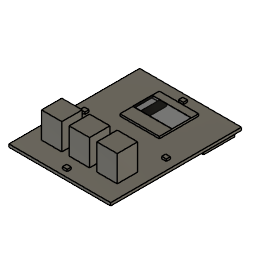
Telemetry Assembly (Autodesk Fusion 360 archive; units mm, degrees)
design "Telemetry PCB"
part number: 2026-03-18-11-21-59-184
Autodesk Fusion 360 part; units mm, degrees
sketch "Sketch1" plane through (0, 0, 0) normal (0, 0, 1) x (1, 0, 0)
  line L0 (-55, 55) -> (15, 55)
  line L1 (15, 55) -> (15, -35)
  line L2 (15, -35) -> (-55, -35)
  line L3 (-55, -35) -> (-55, 55)
  dimension "d1" = 70
  dimension "d2" = 90
  constraint horizontal L0
  constraint vertical L1
  constraint horizontal L2
  constraint vertical L3
  measures "d1" distance of L0.start L0.end
  measures "d2" distance of L0.start L2.end
extrude "Extrude1" add sketch "Sketch1" along normal blind 2 makes body 1
sketch "Display" plane through (0, 0, 2) normal (0, 0, 1) x (-1, 0, 0)
  line L0 (55, 35) -> (-15, 35)
  line L1 (-15, 35) -> (-15, -55)
  line L2 (-15, -55) -> (55, -55)
  line L3 (55, -55) -> (55, 35)
  line L4 (33.31, -46.77) -> (6.31, -46.77)
  line L5 (6.31, -46.77) -> (6.31, -19.77)
  line L6 (6.31, -19.77) -> (33.31, -19.77)
  line L7 (33.31, -19.77) -> (33.31, -46.77)
  line L8 (33.31, -41.77) -> (6.31, -41.77)
  line L9 (6.31, -41.77) -> (6.31, -28.57)
  line L10 (6.31, -28.57) -> (33.31, -28.57)
  line L11 (33.31, -28.57) -> (33.31, -41.77)
  dimension "d5" = 27
  dimension "d6" = 27
  dimension "d7" = 13.2
  dimension "d8" = 5
  dimension "d9" = 8.23
  dimension "d10" = 21.31
  constraint horizontal L4
  constraint vertical L5
  constraint horizontal L6
  constraint vertical L7
  constraint horizontal L8
  constraint vertical L9
  constraint horizontal L10
  constraint vertical L11
  constraint coincident L5 L9.end
  constraint coincident L7 L8.start
  measures "d5" distance of L4.start L4.end
  measures "d6" distance of L4.start L6.end
  measures "d7" distance of L8.start L10.end
  measures "d8" distance of L4 L8
  measures "d9" distance of L2 L4
  measures "d10" distance of L1 L5
extrude "Extrude2" add sketch "Display" along normal blind 1.4 contours L4 L5 L7 L8 | L5 L7 L8 L9 L10 L11 | L5 L6 L7 L10 bodies 1
extrude "Extrude3" add sketch "Display" along normal blind 1.5 contours L5 L7 L8 L9 L10 L11 bodies 1
sketch "Front Instruments" plane through (0, 0, 2) normal (0, 0, 1) x (-1, 0, 0)
  line L0 (21.6, 28.7) -> (18.4, 28.7)
  line L1 (18.4, 28.7) -> (18.4, 31.5)
  line L2 (18.4, 31.5) -> (21.6, 31.5)
  line L3 (21.6, 31.5) -> (21.6, 28.7)
  line L4 (49.6, -8.7) -> (49.6, -11.5)
  line L5 (46.4, -8.7) -> (49.6, -8.7)
  line L6 (49.6, -11.5) -> (46.4, -11.5)
  line L7 (46.4, -11.5) -> (46.4, -8.7)
  line L8 (-6.4, -8.7) -> (-6.4, -11.5)
  line L9 (-9.6, -8.7) -> (-6.4, -8.7)
  line L10 (-6.4, -11.5) -> (-9.6, -11.5)
  line L11 (-9.6, -11.5) -> (-9.6, -8.7)
  line L12 (21.6, -48.387) -> (21.6, -51.187)
  line L13 (18.4, -48.387) -> (21.6, -48.387)
  line L14 (21.6, -51.187) -> (18.4, -51.187)
  line L15 (18.4, -51.187) -> (18.4, -48.387)
  line L16 (-15, 35) -> (-15, -55)
  line L17 (-15, -55) -> (55, -55)
  line L18 (55, 35) -> (-15, 35)
  line L19 (55, -55) -> (55, 35)
  line L20 (27, 7.5) -> (13, 7.5)
  line L21 (13, 7.5) -> (13, 21.5)
  line L22 (13, 21.5) -> (27, 21.5)
  line L23 (27, 21.5) -> (27, 7.5)
  line L24 (46.05, 7.5) -> (32.05, 7.5)
  line L25 (46.05, 21.5) -> (46.05, 7.5)
  line L26 (32.05, 7.5) -> (32.05, 21.5)
  line L27 (32.05, 21.5) -> (46.05, 21.5)
  line L28 (7.95, 7.5) -> (-6.05, 7.5)
  line L29 (7.95, 21.5) -> (7.95, 7.5)
  line L30 (-6.05, 7.5) -> (-6.05, 21.5)
  line L31 (-6.05, 21.5) -> (7.95, 21.5)
  line L32 (-15, 35) -> (55, 35)
  dimension "d15" = 3.2
  dimension "d16" = 2.8
  dimension "d17" = 3.2
  dimension "d18" = 2.8
  dimension "d19" = 3.2
  dimension "d20" = 2.8
  dimension "d21" = 3.2
  dimension "d22" = 2.8
  dimension "d23" = 33.4
  dimension "d24" = 3.813
  dimension "d25" = 33.4
  dimension "d26" = 3.5
  dimension "d27" = 5.4
  dimension "d30" = 5.4
  dimension "d31" = 14
  dimension "d32" = 14
  dimension "d33" = 28
  dimension "d34" = 13.5
  dimension "d35" = 14
  dimension "d36" = 14
  dimension "d37" = 14
  dimension "d38" = 14
  dimension "d65" = 43.7
  dimension "d66" = 43.7
  constraint horizontal L0
  constraint vertical L1
  constraint horizontal L2
  constraint vertical L3
  constraint horizontal L6
  constraint vertical L7
  constraint horizontal L5
  constraint vertical L4
  constraint horizontal L10
  constraint vertical L11
  constraint horizontal L9
  constraint vertical L8
  constraint horizontal L14
  constraint vertical L15
  constraint horizontal L13
  constraint vertical L12
  constraint horizontal L20
  constraint vertical L21
  constraint horizontal L22
  constraint vertical L23
  constraint horizontal L24
  constraint vertical L26
  constraint horizontal L27
  constraint vertical L25
  constraint horizontal L28
  constraint vertical L30
  constraint horizontal L31
  constraint vertical L29
  measures "d15" distance of L0.start L0.end
  measures "d16" distance of L0.start L2.end
  measures "d17" distance of L4.end L6.end
  measures "d18" distance of L4.end L4.start
  measures "d19" distance of L8.end L10.end
  measures "d20" distance of L8.end L8.start
  measures "d21" distance of L12.end L14.end
  measures "d22" distance of L12.end L12.start
  measures "d23" distance of L15 L16
  measures "d24" distance of L14 L17
  measures "d25" distance of L1 L16
  measures "d26" distance of L2 L18
  measures "d27" distance of L11 L16
  measures "d30" distance of L4 L19
  measures "d31" distance of L20.start L20.end
  measures "d32" distance of L20.start L22.end
  measures "d33" distance of L19 L23
  measures "d34" distance of L18 L22
  measures "d35" distance of L24.end L24.start
  measures "d36" distance of L24.start L25.start
  measures "d37" distance of L28.end L28.start
  measures "d38" distance of L28.start L29.start
  measures "d65" distance of L5 L32
  measures "d66" distance of L9 L32
extrude "Extrude4" add sketch "Front Instruments" along normal blind 18 contours L20 L21 L22 L23 | L24 L25 L26 L27 | L28 L29 L30 L31 bodies 1
extrude "Extrude5" add sketch "Front Instruments" along normal blind 1.4 contours L0 L1 L2 L3 | L4 L5 L6 L7 | L8 L9 L10 L11 | L12 L13 L14 L15 bodies 1
sketch "XIAO" plane through (0, 0, 0) normal (0, 0, -1) x (1, 0, 0)
  line L0 (15, 35) -> (-55, 35)
  line L1 (-55, 35) -> (-55, -55)
  line L2 (-55, -55) -> (15, -55)
  line L3 (15, -55) -> (15, 35)
  line L4 (10.5, -54.9) -> (-7.8, -54.9)
  line L5 (-7.8, -54.9) -> (-7.8, -33.4)
  line L6 (-7.8, -33.4) -> (10.5, -33.4)
  line L7 (10.5, -33.4) -> (10.5, -54.9)
  line L8 (6.35, -59.9) -> (-3.65, -59.9)
  line L9 (-3.65, -59.9) -> (-3.65, -54.9)
  line L10 (-3.65, -54.9) -> (6.35, -54.9)
  line L11 (6.35, -54.9) -> (6.35, -59.9)
  dimension "d43" = 18.3
  dimension "d44" = 21.5
  dimension "d46" = 0.1
  dimension "d47" = 4.5
  dimension "d48" = 10
  dimension "d49" = 5
  dimension "d51" = 5
  dimension "d62" = 4.15
  constraint horizontal L4
  constraint vertical L5
  constraint horizontal L6
  constraint vertical L7
  constraint horizontal L8
  constraint vertical L9
  constraint horizontal L10
  constraint vertical L11
  measures "d43" distance of L4.start L4.end
  measures "d44" distance of L4.start L6.end
  measures "d46" distance of L2 L4
  measures "d47" distance of L3 L7
  measures "d48" distance of L8.start L8.end
  measures "d49" distance of L8.end L9.end
  measures "d51" distance of L4 L8
  measures "d62" distance of L7 L11
extrude "Extrude6" add sketch "XIAO" along normal blind 6 contours L4 L5 L6 L7 L10 bodies 1
extrude "Extrude7" add sketch "XIAO" along normal blind 4 separate body contours L2 L8 L9 L11 makes body 2
move_body "Move1" bodies 2 to x (1, 0, 0) y (0, 1, 0) z (0, 0, 1) at (0, 0, -5)
sketch "MPU 6050" plane through (0, 0, 0) normal (0, 0, -1) x (1, 0, 0)
  line L0 (-31.27, -49.7) -> (-46.77, -49.7)
  line L1 (-46.77, -49.7) -> (-46.77, -29.2)
  line L2 (-46.77, -29.2) -> (-31.27, -29.2)
  line L3 (-31.27, -29.2) -> (-31.27, -49.7)
  line L4 (-55, -55) -> (15, -55)
  line L5 (-55, 35) -> (-55, -55)
  dimension "d56" = 20.5
  dimension "d57" = 15.5
  dimension "d58" = 5.3
  dimension "d59" = 8.23
  constraint horizontal L0
  constraint vertical L1
  constraint horizontal L2
  constraint vertical L3
  measures "d56" distance of L0.start L2.end
  measures "d57" distance of L0.start L0.end
  measures "d58" distance of L0 L4
  measures "d59" distance of L1 L5
extrude "Extrude8" add sketch "MPU 6050" along normal blind 6 bodies 1
extrude "Extrude9" add sketch "XIAO" along normal blind 6 contours L4 L5 L6 L7 L10 bodies 1
move_body "Move2" bodies 2 to x (1, 0, 0) y (0, 1, 0) z (0, 0, 1) at (0, -1, 0)
combine "Combine1" operation add target body 2 tool bodies 1
equation "d10 = 34.81 mm - 13.5 mm"
named bodies: "PCB"
